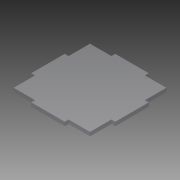
# Autodesk Inventor part: inside_box_front_back
Saved by Autodesk Inventor 2013 (Build 170138000, 138)
## iProperties
Created: 2014-05-23
Part Number: inside_box_front_back
Material: Polycarbonate, Clear
Document SubType Name: Modeling
Designer: balogh
Density: 0.894 g/cm^3
Mass: 9.38262 g
Surface Area: 79.8448 cm^2
Volume: 10.4951 cm^3
Author: balogh
Autodesk Inventor part; units mm, degrees
ref_plane "YZ Plane" through (0, 0, 0) normal (1, 0, 0) x (0, 1, 0)
ref_plane "XZ Plane" through (0, 0, 0) normal (0, 1, 0) x (-1, 0, 0)
ref_plane "XY Plane" through (0, 0, 0) normal (0, 0, 1) x (1, 0, 0)
sketch "Sketch1" plane through (0, 0, 0) normal (0, 0, 1) x (1, 0, 0)
  line L0 (-28.8544, -12.7) -> (-28.8544, -28.8544)
  line L1 (-28.8544, -28.8544) -> (-12.7, -28.8544)
  line L2 (-12.7, -28.8544) -> (-12.7, -31.75)
  line L3 (-12.7, -31.75) -> (12.7, -31.75)
  line L4 (12.7, -31.75) -> (12.7, -28.8544)
  line L5 (12.7, -28.8544) -> (28.8544, -28.8544)
  line L6 (28.8544, -28.8544) -> (28.8544, -12.7)
  line L7 (28.8544, -12.7) -> (31.75, -12.7)
  line L8 (31.75, -12.7) -> (31.75, 12.7)
  line L9 (31.75, 12.7) -> (28.8544, 12.7)
  line L10 (28.8544, 12.7) -> (28.8544, 28.8544)
  line L11 (28.8544, 28.8544) -> (12.7, 28.8544)
  line L12 (12.7, 28.8544) -> (12.7, 31.75)
  line L13 (12.7, 31.75) -> (-12.7, 31.75)
  line L14 (-12.7, 31.75) -> (-12.7, 28.8544)
  line L15 (-12.7, 28.8544) -> (-28.8544, 28.8544)
  line L16 (-28.8544, 28.8544) -> (-28.8544, 12.7)
  line L17 (-28.8544, 12.7) -> (-31.75, 12.7)
  line L18 (-31.75, 12.7) -> (-31.75, -12.7)
  line L19 (-31.75, -12.7) -> (-28.8544, -12.7)
  point P0 (0, 0)
  constraints: 40 end point, 10 parallel, 6 perpendicular, 3 collinear
extrude "Extrusion1" add sketch "Sketch1" along normal blind 2.8956
body "Solid1"
